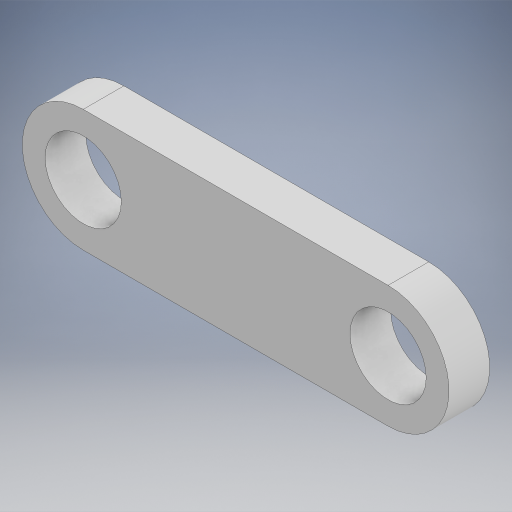
# Autodesk Inventor part: CE-9.3.2-crank
Saved by Autodesk Inventor 2024 (Build 280153000, 153)
## iProperties
Created: 2024-03-22
Part Number: CE-9.3.2-crank
Material: Generic
Document SubType Name: Modeling
Designer: Alex
Density: 1 g/cm^3
Appearance: Default
Author: Alex
Autodesk Inventor part; units mm, degrees
ref_plane "YZ Plane" through (0, 0, 0) normal (1, 0, 0) x (0, 1, 0)
ref_plane "XZ Plane" through (0, 0, 0) normal (0, 1, 0) x (-1, 0, 0)
ref_plane "XY Plane" through (0, 0, 0) normal (0, 0, 1) x (1, 0, 0)
sketch "Sketch1" plane through (0, 0, 0) normal (0, 0, 1) x (1, 0, 0)
  line L0 (-30, 0) -> (30, 0) construction
  line L1 (-30, 12) -> (30, 12)
  line L2 (30, -12) -> (-30, -12)
  arc A0 (-30, 12) -> (-30, -12) centre (-30, 0) ccw
  arc A1 (30, -12) -> (30, 12) centre (30, 0) ccw
  circle A2 centre (-30, 0) radius 7.5
  circle A3 centre (30, 0) radius 7.5
  point P0 (0, 0)
  dimension "d0" = 60
  dimension "d1" = 12
  dimension "d2" = 15
  constraints: 8 end point, 4 centre point, 4 point on circle, 4 tangent, 2 coincident, 1 equal radius, 1 horizontal, 1 midpoint, 1 parallel
  measures "d0" distance of L1.start L1.end
  measures "d1" radius of A1
  measures "d2" diameter of A2
extrude "Extrusion1" add sketch "Sketch1" along normal mid plane 8
body "Solid1"
